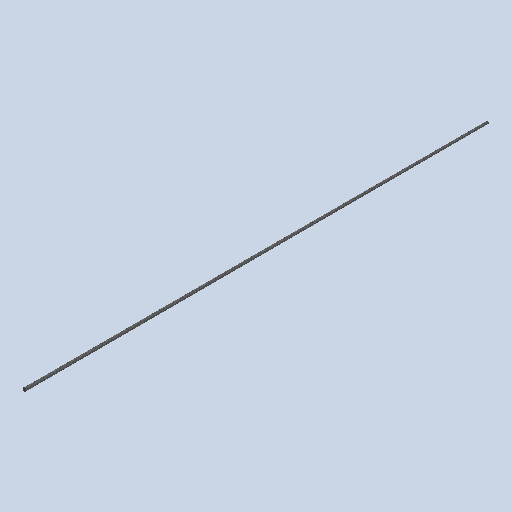
# Autodesk Inventor part: Rear Wing Spar (tapered solid)
Saved by Autodesk Inventor 2025.1 (Build 291241000, 241)
## iProperties
Category: <PART CATAGORY>
Created: 2024-11-15
Part Number: Rear Wing Spar (tapered solid)
Material: CFRP
Document SubType Name: Modeling
Designer: chowg
Density: 1.43 g/cm^3
Appearance: Carbon Fiber
Title: <TITLE>
Author: chowg
Revision Number: 1
Autodesk Inventor part; units mm, degrees
ref_plane "YZ Plane" through (0, 0, 0) normal (1, 0, 0) x (0, 1, 0)
ref_plane "XZ Plane" through (0, 0, 0) normal (0, 1, 0) x (-1, 0, 0)
ref_plane "XY Plane" through (0, 0, 0) normal (0, 0, 1) x (1, 0, 0)
sketch "Sketch6" plane through (0, 0, 0) normal (1, 0, 0) x (0, 1, 0)
  line L0 (0, 0) -> (4, 0)
  line L1 (0, 0) -> (4, 0) construction
  line L2 (0, 0) -> (0, -1200)
  line L3 (0, 0) -> (1200, 0) construction
  line L4 (0, -1200) -> (3, -1200)
  line L5 (3, -1200) -> (4, 0)
  dimension "d85" = 4
  dimension "d86" = 0
  dimension "d87" = 1200
  dimension "d88" = 90
  dimension "d89" = 3
  dimension "d90" = 90
  constraints: 12 end point, 3 horizontal, 2 equal length, 2 perpendicular
  measures "d85" distance of L0.start L0.end
  measures "d86" distance between parallel lines of L0 L1
  measures "d87" distance of L0.start L2.end
  measures "d88" angle of L2 L3
  measures "d89" distance of L2.end L4.end
  measures "d90" angle of L4 L2
revolve "Revolution1" add sketch "Sketch6" angle 360 about axis through (0, 0, 0) along (0, 0, -1)
body "Solid2"
